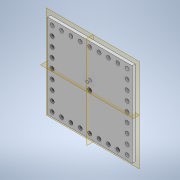
# Autodesk Inventor part: MessHalterV2
Saved by Autodesk Inventor 2021 (Build 250183000, 183)
## iProperties
Created: 2020-06-29
Part Number: MessHalterV2
Material: Generisch
Document SubType Name: Modeling
Designer: marvi
Density: 1 g/cm^3
Appearance: Vorgabe
Author: marvi
Autodesk Inventor part; units mm, degrees
sketch "Skizze1" plane through (0, 0, 0) normal (0, 0, 1) x (1, 0, 0)
  line L0 (-70, 70) -> (70, 70)
  line L1 (70, 70) -> (70, -70)
  line L2 (70, -70) -> (-70, -70)
  line L3 (-70, -70) -> (-70, 70)
  line L4 (0, 98) -> (0, -98) projected
  line L5 (-98, 0) -> (98, 0) projected
  point P0 (0, 0)
  dimension "d0" = 70
  dimension "d1" = 140
  dimension "d2" = 140
  dimension "d3" = 70
  constraints: 8 end point, 2 parallel, 1 horizontal, 1 perpendicular
  measures "d0" distance between parallel lines of L4 L3
  measures "d1" distance of L0.start L0.end
  measures "d2" distance of L2.end L0.start
  measures "d3" distance between parallel lines of L0 L5
extrude "Extrusion1" add sketch "Skizze1" along normal blind 5
sketch "Skizze2" plane through (0, 0, 5) normal (0, 0, 1) x (1, 0, 0)
  point P0 (0, 0)
  point P1 (0, 0)
  constraints: 1 coincident
hole "Bohrung1" at (0, 0, 5) direction (0, 0, -1) diameter 6.7 depth 9.5
sketch "Skizze3" plane through (0, 0, 5) normal (0, 0, 1) x (1, 0, 0)
  circle A0 centre (0, 0) radius 3.35 projected
  circle A1 centre (0, 0) radius 3.35 projected
  line L0 (-70, 70) -> (-70, -70) projected
  line L1 (-70, -70) -> (70, -70) projected
  line L2 (70, -70) -> (70, 70) projected
  line L3 (70, 70) -> (-70, 70) projected
  circle A2 centre (0, 14) radius 2.35
  dimension "d13" = 14
  dimension "d14" = 4.7
  constraints: 1 centre point, 1 coincident
  measures "d13" distance of point (0, 14) A0.centre
  measures "d14" diameter of A2
extrude "Extrusion2" add sketch "Skizze3" along normal blind 4.3 contours A2
sketch "Skizze4" plane through (0, 0, 5) normal (0, 0, 1) x (1, 0, 0)
  circle A0 centre (0, 14) radius 2.35 projected
  circle A1 centre (0, 0) radius 3.35 projected
  line L0 (-70, 70) -> (-70, -70) projected
  line L1 (-70, -70) -> (70, -70) projected
  line L2 (70, -70) -> (70, 70) projected
  line L3 (70, 70) -> (-70, 70) projected
  line L4 (-98, 0) -> (98, 0) projected
  line L5 (0, 98) -> (0, -98) projected
  point P0 (-62, 62)
  point P1 (62, 62)
  point P2 (-62, -62)
  point P3 (62, -62)
  dimension "d17" = 62
  dimension "d18" = 62
  dimension "d21" = 124
  dimension "d24" = 124
  constraints: 1 horizontal, 1 vertical, 3 other
  measures "d17" distance from line of point (-62, 62) L4
  measures "d18" distance from line of point (-62, 62) L5
  measures "d21" distance of point (-62, 62) point (62, 62)
  measures "d24" distance of point (-62, 62) point (-62, -62)
hole "Bohrung2" at (-62, 62, 5) at (62, 62, 5) at (-62, -62, 5) at (62, -62, 5) direction (0, 0, -1) diameter 6.3 end through all
sketch "Skizze5" plane through (0, 0, 5) normal (0, 0, 1) x (1, 0, 0)
  circle A0 centre (-62, -62) radius 3.15 projected
  circle A1 centre (-62, 62) radius 3.15 projected
  circle A2 centre (62, 62) radius 3.15 projected
  circle A3 centre (62, -62) radius 3.15 projected
  circle A4 centre (0, 14) radius 2.35 projected
  circle A5 centre (0, 0) radius 3.35 projected
  line L0 (-70, 70) -> (-70, -70) projected
  line L1 (-70, -70) -> (70, -70) projected
  line L2 (70, -70) -> (70, 70) projected
  line L3 (70, 70) -> (-70, 70) projected
  line L4 (0, 98) -> (0, -98) projected
  line L5 (-98, 0) -> (98, 0) projected
  point P0 (-62, 0)
  point P1 (-62, 15.5)
  point P2 (-62, 31)
  point P3 (-62, 46.5)
  point P4 (0, 62)
  point P5 (-15.5, 62)
  point P6 (-31, 62)
  point P7 (-46.5, 62)
  dimension "d35" = 62
  dimension "d36" = 0
  dimension "d37" = 15.5
  dimension "d38" = 15.5
  dimension "d39" = 15.5
  dimension "d40" = 15.5
  dimension "d41" = 31
  dimension "d42" = 46.5
  constraints: 1 point on line
  measures "d35" distance from line of point (-62, 0) L4
  measures "d36" distance from line of L5 point (-62, 0)
  measures "d37" distance of point (-62, 15.5) point (-62, 0)
  measures "d38" distance of point (-62, 31) point (-62, 15.5)
  measures "d39" distance of point (-62, 46.5) point (-62, 31)
  measures "d40" distance from line of point (-15.5, 62) L4
  measures "d41" distance from line of L4 point (-31, 62)
  measures "d42" distance from line of L4 point (-46.5, 62)
hole "Bohrung3" at (-62, 0, 5) at (-62, 15.5, 5) at (-62, 31, 5) at (-62, 46.5, 5) at (0, 62, 5) at (-15.5, 62, 5) at (-31, 62, 5) at (-46.5, 62, 5) direction (0, 0, -1) diameter 6.3 end through all
mirror "Spiegeln1" about plane through (0, 0, 0) normal (1, 0, 0) of "Bohrung3"
mirror "Spiegeln2" about plane through (0, 0, 0) normal (0, 1, 0) of "Bohrung3", "Spiegeln1"
equation "\"d0\" = 0.5 * d1"
equation "\"d3\" = 0.5 * d2"
